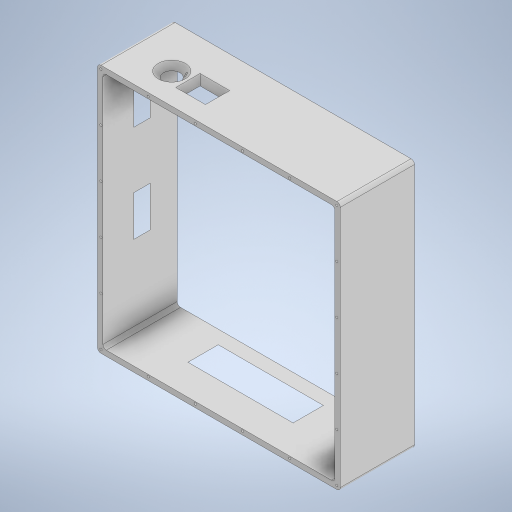
# Autodesk Inventor part: middle
Saved by Autodesk Inventor 2024 (Build 280153000, 153)
## iProperties
Created: 2023-05-28
Part Number: middle
Material: Generic
Document SubType Name: Modeling
Designer: elect
Density: 1 g/cm^3
Appearance: Default
Author: elect
Autodesk Inventor part; units mm, degrees
ref_plane "YZ Plane" through (0, 0, 0) normal (1, 0, 0) x (0, 1, 0)
ref_plane "XZ Plane" through (0, 0, 0) normal (0, 1, 0) x (-1, 0, 0)
ref_plane "XY Plane" through (0, 0, 0) normal (0, 0, 1) x (1, 0, 0)
sketch "Sketch1" plane through (0, 0, 0) normal (0, 0, 1) x (1, 0, 0)
  line L0 (-116.0602, 124.2038) -> (96.0298, 124.2038)
  line L1 (99.2048, 121.0288) -> (99.2048, -97.4112)
  line L2 (96.0298, -100.5862) -> (-116.0602, -100.5862)
  line L3 (-119.2352, -97.4112) -> (-119.2352, 121.0288)
  line L4 (-121.1402, 129.2838) -> (101.1098, 129.2838)
  line L5 (104.2848, 126.1088) -> (104.2848, -102.4912)
  line L6 (101.1098, -105.6662) -> (-121.1402, -105.6662)
  line L7 (-124.3152, -102.4912) -> (-124.3152, 126.1088)
  arc A0 (-121.1402, 129.2838) -> (-124.3152, 126.1088) centre (-121.1402, 126.1088) ccw
  arc A1 (-116.0602, 124.2038) -> (-119.2352, 121.0288) centre (-116.0602, 121.0288) ccw
  arc A2 (-124.3152, -102.4912) -> (-121.1402, -105.6662) centre (-121.1402, -102.4912) ccw
  arc A3 (-119.2352, -97.4112) -> (-116.0602, -100.5862) centre (-116.0602, -97.4112) ccw
  arc A4 (101.1098, -105.6662) -> (104.2848, -102.4912) centre (101.1098, -102.4912) ccw
  arc A5 (96.0298, -100.5862) -> (99.2048, -97.4112) centre (96.0298, -97.4112) ccw
  arc A6 (99.2048, 121.0288) -> (96.0298, 124.2038) centre (96.0298, 121.0288) ccw
  arc A7 (104.2848, 126.1088) -> (101.1098, 129.2838) centre (101.1098, 126.1088) ccw
  point P0 (0, 0)
  point P1 (104.2848, -105.6662)
  point P2 (104.2848, 129.2838)
  point P3 (-124.3152, -105.6662)
  dimension "d0" = 234.95
  dimension "d1" = 228.6
  dimension "d2" = 5.08
  dimension "d3" = 5.08
  dimension "d4" = 5.08
  dimension "d5" = 5.08
  dimension "d6" = 3.175
  constraints: 16 end point, 16 point on circle, 16 tangent, 8 centre point, 7 equal radius, 6 point on line, 4 parallel, 2 horizontal, 2 perpendicular
  measures "d0" distance of point (104.285, 129.284) point (104.285, -105.666)
  measures "d1" distance of point (104.285, -105.666) point (-124.315, -105.666)
  measures "d2" distance between parallel lines of L6 L2
  measures "d3" distance between parallel lines of L3 L7
  measures "d4" distance between parallel lines of L0 L4
  measures "d5" distance between parallel lines of L5 L1
  measures "d6" radius of A0
extrude "Extrusion1" add sketch "Sketch1" along normal blind 69.85
sketch "Sketch2" plane through (0, 0, 69.85) normal (0, 0, 1) x (1, 0, 0)
  arc A0 (-121.1402, 129.2838) -> (-124.3152, 126.1088) centre (-121.1402, 126.1088) ccw projected
  line L0 (-119.2352, -97.4112) -> (-119.2352, 121.0288) projected
  line L1 (-116.0602, 124.2038) -> (96.0298, 124.2038) projected
  point P0 (0, 0)
  point P1 (-121.1402, 80.3888)
  point P2 (-121.1402, 34.6688)
  point P3 (-121.1402, -11.0512)
  point P4 (-121.1402, -56.7712)
  point P5 (-121.1402, -102.4912)
  point P6 (-76.6902, -102.4912)
  point P7 (-32.2402, -102.4912)
  point P8 (12.2098, -102.4912)
  point P9 (56.6598, -102.4912)
  point P10 (101.1098, -102.4912)
  point P11 (-76.6902, 126.1088)
  point P12 (-32.2402, 126.1088)
  point P13 (12.2098, 126.1088)
  point P14 (56.6598, 126.1088)
  point P15 (101.1098, 126.1088)
  point P16 (101.1098, 80.3888)
  point P17 (101.1098, 34.6688)
  point P18 (101.1098, -11.0512)
  point P19 (101.1098, -56.7712)
  dimension "d11" = 45.72
  dimension "d18" = 44.45
  dimension "d25" = 44.45
  dimension "d32" = 45.72
  constraints: 2 horizontal, 2 vertical, 1 coincident, 19 other
  measures "d11" distance of point (-121.14, 126.109) point (-121.14, 80.389)
  measures "d18" distance of point (-121.14, -102.491) point (-76.69, -102.491)
  measures "d25" distance of point (-121.14, 126.109) point (-76.69, 126.109)
  measures "d32" distance of point (101.11, 126.109) point (101.11, 80.389)
hole "Hole1" at (-121.1402, 126.1088, 69.85) at (-121.1402, 80.3888, 69.85) at (-121.1402, 34.6688, 69.85) at (-121.1402, -11.0512, 69.85) at (-121.1402, -56.7712, 69.85) at (-121.1402, -102.4912, 69.85) at (-76.6902, -102.4912, 69.85) at (-32.2402, -102.4912, 69.85) at (12.2098, -102.4912, 69.85) at (56.6598, -102.4912, 69.85) at (101.1098, -102.4912, 69.85) at (-76.6902, 126.1088, 69.85) at (-32.2402, 126.1088, 69.85) at (12.2098, 126.1088, 69.85) at (56.6598, 126.1088, 69.85) at (101.1098, 126.1088, 69.85) at (101.1098, 80.3888, 69.85) at (101.1098, 34.6688, 69.85) at (101.1098, -11.0512, 69.85) at (101.1098, -56.7712, 69.85) direction (0, 0, -1) diameter 2.032 end through all
sketch "Sketch3" plane through (99.2048, -97.4112, 0) normal (-1, 0, 0) x (0, 0, 1)
  circle A0 centre (12.7, 42.545) radius 3
  circle A1 centre (57.15, 42.545) radius 3
  circle A2 centre (57.15, 137.795) radius 3
  circle A3 centre (12.7, 137.795) radius 3
  line L0 (69.85, -5.08) -> (69.85, 223.52) projected
  line L1 (0, -5.08) -> (0, 223.52) projected
  line L2 (0, -8.255) -> (69.85, -8.255) projected
  point P0 (0, 97.4112)
  dimension "d44" = 95.25
  dimension "d45" = 6
  dimension "d46" = 44.45
  dimension "d47" = 12.7
  dimension "d48" = 12.7
  dimension "d49" = 50.8
  constraints: 4 centre point, 3 equal radius, 2 horizontal alignment, 2 vertical alignment
  measures "d44" distance of A1.centre A2.centre
  measures "d45" diameter of A2
  measures "d46" distance of A2.centre A3.centre
  measures "d47" distance from line of L0 A2.centre
  measures "d48" distance from line of L1 A3.centre
  measures "d49" distance from line of L2 A1.centre
extrude "Extrusion2" add sketch "Sketch3" along normal blind 6.35
sketch "Sketch4" plane through (92.8548, 40.3838, 12.7) normal (-1, 0, 0) x (0, 0, 1)
  circle A0 centre (0, 0) radius 3 projected
  circle A1 centre (44.45, 0) radius 3 projected
  circle A2 centre (0, -95.25) radius 3 projected
  circle A3 centre (44.45, -95.25) radius 3 projected
  point P0 (-12.7, -40.3838)
  constraints: 4 coincident
hole "Hole2" at (92.8548, 40.3838, 12.7) at (92.8548, 40.3838, 57.15) at (92.8548, -54.8662, 12.7) at (92.8548, -54.8662, 57.15) direction (1, 0, 0) diameter 2.75 depth 6.35 tip angle 118
sketch "Sketch5" plane through (-121.1402, -105.6662, 0) normal (0, -1, 0) x (1, 0, 0)
  line L0 (53.34, 41.275) -> (152.4, 41.275)
  line L1 (152.4, 41.275) -> (152.4, 12.7)
  line L2 (152.4, 12.7) -> (53.34, 12.7)
  line L3 (53.34, 12.7) -> (53.34, 41.275)
  line L4 (0, 0) -> (222.25, 0) projected
  line L5 (0, 69.85) -> (222.25, 69.85) projected
  line L6 (222.25, 0) -> (222.25, 69.85) projected
  line L7 (0, 0) -> (0, 69.85) projected
  point P0 (121.1402, 0)
  point P1 (53.34, 26.9875)
  dimension "d59" = 12.7
  dimension "d60" = 28.575
  dimension "d61" = 69.85
  dimension "d62" = 53.34
  constraints: 8 end point, 2 parallel, 1 horizontal, 1 midpoint, 1 perpendicular
  measures "d59" distance between parallel lines of L4 L2
  measures "d60" distance between parallel lines of L5 L0
  measures "d61" distance between parallel lines of L6 L1
  measures "d62" distance from line of L7 point (53.34, 26.987)
extrude "Extrusion3" cut sketch "Sketch5" against normal blind 6.35 contours L0 L1 L2 L3
sketch "Sketch6" plane through (-67.8002, -105.6662, 12.7) normal (0, 0, 1) x (1, 0, 0)
  circle A0 centre (35.56, 3.175) radius 1.016 projected
  circle A1 centre (80.01, 3.175) radius 1.016 projected
  point P0 (67.8002, 105.6662)
extrude "Extrusion4" add sketch "Sketch6" against normal blind 3.175
sketch "Sketch7" plane through (31.2598, -105.6662, 41.275) normal (0, 0, -1) x (-1, 0, 0)
  circle A0 centre (63.5, 3.175) radius 1.016 projected
  circle A1 centre (19.05, 3.175) radius 1.016 projected
  point P0 (31.2598, 105.6662)
extrude "Extrusion5" add sketch "Sketch7" against normal blind 3.175
chamfer "Chamfer1" distance 5.08 angle 45 4 edges at (-18.2702, -105.6662, 12.7) (-67.8002, -105.6662, 26.9875) (-18.2702, -105.6662, 41.275) (31.2598, -105.6662, 26.9875)
sketch "Sketch8" plane through (-124.3152, -102.4912, 0) normal (-1, 0, 0) x (0, 0, 1)
  line L0 (40.64, 205.74) -> (25.4, 205.74)
  line L1 (25.4, 205.74) -> (25.4, 167.64)
  line L2 (25.4, 167.64) -> (40.64, 167.64)
  line L3 (40.64, 167.64) -> (40.64, 205.74)
  line L4 (40.64, 114.3) -> (25.4, 114.3)
  line L5 (25.4, 114.3) -> (25.4, 76.2)
  line L6 (25.4, 76.2) -> (40.64, 76.2)
  line L7 (40.64, 76.2) -> (40.64, 114.3)
  line L8 (0, 228.6) -> (0, 0) projected
  line L9 (0, 228.6) -> (69.85, 228.6) projected
  point P0 (0, 102.4912)
  point P1 (33.02, 205.74)
  point P2 (33.02, 114.3)
  dimension "d73" = 25.4
  dimension "d74" = 25.4
  dimension "d75" = 22.86
  dimension "d76" = 53.34
  dimension "d77" = 38.1
  dimension "d78" = 38.1
  dimension "d81" = 15.24
  dimension "d82" = 15.24
  constraints: 16 end point, 5 equal length, 2 horizontal, 2 midpoint, 2 perpendicular
  measures "d73" distance between parallel lines of L8 L1
  measures "d74" distance between parallel lines of L8 L5
  measures "d75" distance from line of L9 point (33.02, 205.74)
  measures "d76" distance from line of point (33.02, 114.3) L2
  measures "d77" distance of L2.end L0.start
  measures "d78" distance of L6.end L4.start
  measures "d81" distance of L0.start L0.end
  measures "d82" distance of L4.start L4.end
extrude "Extrusion6" cut sketch "Sketch8" against normal up to surface (5.08 mm away)
sketch "Sketch9" plane through (-124.3152, 65.1488, 25.4) normal (0, 0, 1) x (1, 0, 0)
  circle A0 centre (3.175, 15.24) radius 1.016 projected
  circle A1 centre (3.175, -76.2) radius 1.016 projected
  circle A2 centre (3.175, -76.2) radius 1.016 projected
  line L0 (0, 38.1) -> (0, 0) projected
  circle A3 centre (3.175, 15.24) radius 1.016 projected
  point P0 (124.3152, -65.1488)
extrude "Extrusion7" add sketch "Sketch9" against normal blind 3.175
sketch "Sketch11" plane through (-124.3152, 65.1488, 40.64) normal (0, 0, -1) x (-1, 0, 0)
  circle A0 centre (-3.175, 15.24) radius 1.016 projected
  circle A1 centre (-3.175, -76.2) radius 1.016 projected
  point P0 (-124.3152, -65.1488)
extrude "Extrusion8" add sketch "Sketch11" against normal blind 3.175
chamfer "Chamfer2" distance 5.08 angle 45 8 edges at (-124.3152, 84.1988, 40.64) (-124.3152, 103.2488, 33.02) (-124.3152, 84.1988, 25.4) (-124.3152, 65.1488, 33.02) (-124.3152, 11.8088, 33.02) (-124.3152, -7.2412, 40.64) (-124.3152, -7.2412, 25.4) (-124.3152, -26.2912, 33.02)
sketch "Sketch12" plane through (-121.1402, 129.2838, 0) normal (0, 1, 0) x (1, 0, 0)
  circle A0 centre (38.1, -41.275) radius 7.62
  line L0 (152.4, -41.275) -> (53.34, -41.275) projected
  line L1 (0, 0) -> (0, -69.85) projected
  line L2 (222.25, -69.85) -> (0, -69.85) projected
  line L3 (76.2, -47.625) -> (58.42, -47.625)
  line L4 (58.42, -47.625) -> (58.42, -34.925)
  line L5 (58.42, -34.925) -> (76.2, -34.925)
  line L6 (76.2, -34.925) -> (76.2, -47.625)
  point P0 (121.1402, 0)
  point P1 (58.42, -41.275)
  dimension "d90" = 15.24
  dimension "d94" = 38.1
  dimension "d95" = 28.575
  dimension "d96" = 12.7
  dimension "d97" = 17.78
  dimension "d98" = 20.32
  constraints: 8 end point, 2 parallel, 1 centre point, 1 horizontal, 1 horizontal alignment, 1 midpoint, 1 perpendicular
  measures "d90" diameter of A0
  measures "d94" distance from line of L1 A0.centre
  measures "d95" distance from line of L2 A0.centre
  measures "d96" distance of L5.end L3.start
  measures "d97" distance of L3.start L3.end
  measures "d98" distance from line of A0.centre L4
extrude "Extrusion9" cut sketch "Sketch12" against normal up to surface (5.08 mm away)
chamfer "Chamfer4" distance 5.08 angle 45 5 edges at (-53.8302, 129.2838, 47.625) (-44.9402, 129.2838, 41.275) (-53.8302, 129.2838, 34.925) (-62.7202, 129.2838, 41.275) (-90.6602, 129.2838, 41.275)
body "Solid1"
